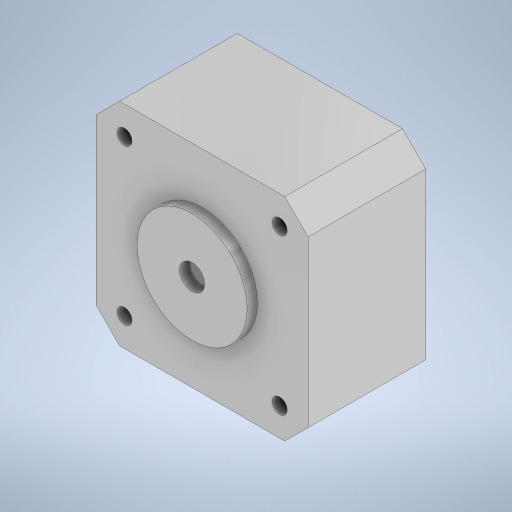
# Autodesk Inventor part: Мотор
Saved by Autodesk Inventor 2024 (Build 280153020, 153B)
## iProperties
Created: 2023-02-23
Part Number: Мотор
Material: Типовые
Document SubType Name: Modeling
Designer: Admin
Density: 1 g/cm^3
Appearance: По умолчанию
Author: Admin
Autodesk Inventor part; units mm, degrees
ref_plane "YZ Plane" through (0, 0, 0) normal (1, 0, 0) x (0, 1, 0)
ref_plane "XZ Plane" through (0, 0, 0) normal (0, 1, 0) x (-1, 0, 0)
ref_plane "XY Plane" through (0, 0, 0) normal (0, 0, 1) x (1, 0, 0)
sketch "Эскиз1" plane through (0, 0, 0) normal (0, 0, 1) x (1, 0, 0)
  line L0 (-21.15, -21.15) -> (21.15, -21.15)
  line L1 (21.15, -21.15) -> (21.15, 21.15)
  line L2 (21.15, 21.15) -> (-21.15, 21.15)
  line L3 (-21.15, 21.15) -> (-21.15, -21.15)
  line L4 (-21.15, -21.15) -> (21.15, 21.15) construction
  line L5 (21.15, -21.15) -> (-21.15, 21.15) construction
  circle A0 centre (-15.5, 15.5) radius 1.5
  line L6 (0, 0) -> (0, 3.5329)
  line L7 (0, 0) -> (3.0649, 0)
  circle A1 centre (15.5, 15.5) radius 1.5
  circle A2 centre (15.5, -15.5) radius 1.5
  circle A3 centre (-15.5, -15.5) radius 1.5
  line L8 (-8.1, -21.15) -> (8.1, -21.15)
  line L9 (8.1, -21.15) -> (8.1, -26.65)
  line L10 (8.1, -26.65) -> (-8.1, -26.65)
  line L11 (-8.1, -26.65) -> (-8.1, -21.15)
  point P0 (0, -26.65)
  dimension "d3" = 42.3
  dimension "d7" = 3
  dimension "d11" = 31
  dimension "d12" = 31
  dimension "d13" = 16.2
  dimension "d14" = 5.5
  constraints: 24 end point, 4 centre point, 4 parallel, 3 horizontal, 3 midpoint, 3 perpendicular, 3 symmetric about line, 1 point on line, 1 vertical, 1 vertical alignment, 3 other
  measures "d3" distance of L1.end L2.end
  measures "d7" diameter of A0
  measures "d11" distance of A3.centre A0.centre
  measures "d12" distance of A2.centre A3.centre
  measures "d13" distance of L9.end L10.end
  measures "d14" distance of L8.end L9.end
extrude "Выдавливание1" add sketch "Эскиз1" along normal blind 9.2 contours L0 L9 L10 L11
extrude "Выдавливание2" add sketch "Эскиз1" along normal blind 23.5 contours L3 L2 L1 L0
sketch "Эскиз2" plane through (0, 0, 23.5) normal (0, 0, 1) x (1, 0, 0)
  circle A0 centre (0, 0) radius 11
  circle A1 centre (0, 0) radius 2.5
  line L0 (-1.5, 2) -> (1.5, 2)
  point P0 (0, 2)
  dimension "d19" = 22
  dimension "d20" = 5
  dimension "d21" = 4.5
  constraints: 2 centre point, 2 coincident, 2 end point, 2 point on circle, 1 horizontal, 1 midpoint, 1 vertical alignment
  measures "d19" diameter of A0
  measures "d20" diameter of A1
extrude "Выдавливание3" add sketch "Эскиз2" along normal blind 2
extrude "Выдавливание4" add sketch "Эскиз2" along normal blind 22 separate body contours A1 L0 picked at (0.1119, 0.5076)
chamfer "Фаска1" distance 4.65 angle 45 4 edges at (-21.15, 21.15, 11.75) (21.15, 21.15, 11.75) (-21.15, -21.15, 11.75) (21.15, -21.15, 11.75)
